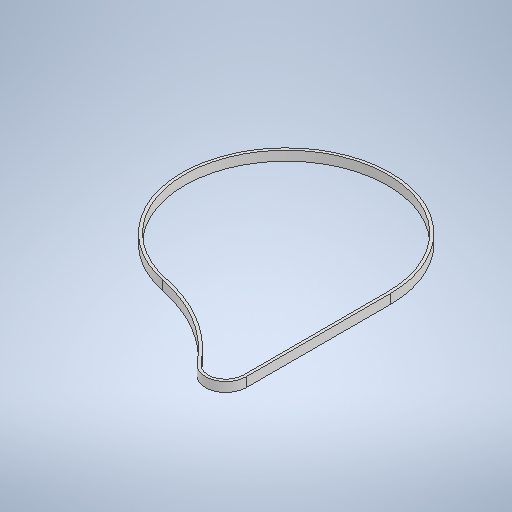
# Autodesk Inventor part: 50-01-002
Saved by Autodesk Inventor 2025.2 (Build 292293000, 293)
## iProperties
Created: 2024-11-29
Part Number: 50-01-002
Material: Generic
Document SubType Name: Modeling
Designer: Zvonko.Gabric
Density: 1 g/cm^3
Appearance: Default
Author: Zvonko.Gabric
Autodesk Inventor part; units mm, degrees
ref_plane "YZ Plane" through (0, 0, 0) normal (1, 0, 0) x (0, 1, 0)
ref_plane "XZ Plane" through (0, 0, 0) normal (0, 1, 0) x (-1, 0, 0)
ref_plane "XY Plane" through (0, 0, 0) normal (0, 0, 1) x (1, 0, 0)
sketch "Sketch1" plane through (0, 0, 0) normal (0, 1, 0) x (-1, 0, 0)
  line L0 (-74.3921, 163.9674) -> (-70.2288, 159.0593)
  line L1 (-107, 0) -> (-107, 152)
  line L2 (-67.941, 161) -> (-72.1044, 165.9081)
  line L3 (-110, 152) -> (-110, 0)
  arc A0 (-107, 0) -> (21.4, 104.8382) centre (0, 0) ccw
  arc A1 (-70.2288, 159.0593) -> (21.4, 104.8382) centre (53.9741, 264.418) ccw
  arc A2 (-74.3921, 163.9674) -> (-107, 152) centre (-88.5, 152) ccw
  arc A3 (-72.1044, 165.9081) -> (-110, 152) centre (-88.5, 152) ccw
  arc A4 (-67.941, 161) -> (22, 107.7775) centre (53.9741, 264.418) ccw
  arc A5 (-110, 0) -> (22, 107.7775) centre (0, 0) ccw
  dimension "d0" = 0
  dimension "d1" = 110
  dimension "d2" = 107
  dimension "d3" = 175.887
  dimension "d4" = 18.5
  dimension "d5" = 21.5
  dimension "d6" = 159.8705
  dimension "d7" = 162.8705
  dimension "d8" = 269.8705
  dimension "d9" = 152
  dimension "d10" = 152
  dimension "d11" = 88.5
  dimension "d12" = 3
  constraints: 12 point on circle, 8 end point, 6 centre point
  measures "d0" distance of point (0, 0) A0.centre
  measures "d1" radius of A5
  measures "d2" radius of A0
  measures "d3" distance of point (0, 0) A2.centre
  measures "d4" radius of A2
  measures "d5" radius of A3
  measures "d6" radius of A4
  measures "d7" radius of A1
  measures "d8" distance of point (0, 0) A1.centre
  measures "d9" distance of L1.start L1.end
  measures "d10" distance of L3.start L3.end
  measures "d11" horizontal distance of point (0, 0) A2.centre
  measures "d12" distance between parallel lines of L3 L1
extrude "Extrusion1" add sketch "Sketch1" along normal blind 10
body "Solid1"
